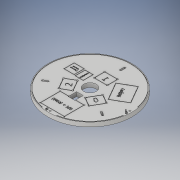
# Autodesk Inventor part: Robot Plate v1.4
Saved by Autodesk Inventor 2019 (Build 230136000, 136)
## iProperties
Created: 2019-02-04
Part Number: Robot Plate v1.4
Material: Generic
Document SubType Name: Modeling
Designer: a1213969
Density: 1 g/cm^3
Appearance: Default
Author: a1213969
Autodesk Inventor part; units mm, degrees
(part 1 of 4)
ref_plane "YZ Plane" through (0, 0, 0) normal (1, 0, 0) x (0, 1, 0)
ref_plane "XZ Plane" through (0, 0, 0) normal (0, 1, 0) x (-1, 0, 0)
ref_plane "XY Plane" through (0, 0, 0) normal (0, 0, 1) x (1, 0, 0)
sketch "Sketch1" plane through (0, 0, 0) normal (0, 1, 0) x (-1, 0, 0)
  circle A0 centre (0, 0) radius 100
  circle A1 centre (0, 0) radius 15
  dimension "d0" = 200
  dimension "d1" = 30
  constraints: 2 centre point, 2 coincident
  measures "d0" diameter of A0
  measures "d1" diameter of A1
extrude "Extrusion1" add sketch "Sketch1" along normal blind 10
sketch "Sketch2" plane through (0, 10, 0) normal (0, 1, 0) x (1, 0, 0)
  circle A0 centre (0, 0) radius 15 construction
  circle A1 centre (0, 0) radius 100 construction
  line L0 (140, 0) -> (-140, 0) construction
  line L1 (0, 140) -> (0, -140) construction
  line L2 (0, 0) -> (0, 38) construction
  line L3 (15, 26) -> (-15, 26) construction
  line L4 (-15, 26) -> (-15, 50) construction
  line L5 (-15, 50) -> (15, 50) construction
  line L6 (15, 50) -> (15, 26) construction
  line L7 (15, 26) -> (-15, 50) construction
  line L8 (-15, 26) -> (15, 50) construction
  dimension "d4" = 38
  dimension "d5" = 30
  dimension "d6" = 24
  constraints: 14 end point, 4 coincident, 2 midpoint, 2 parallel, 1 horizontal, 1 perpendicular, 1 point on line
  measures "d4" distance of L2.start L2.end
  measures "d5" distance of L4.end L5.end
  measures "d6" distance between parallel lines of L3 L5
hole "Hole1" at (15, 10, -50) at (-15, 10, -26) at (-15, 10, -50) at (15, 10, -50) at (-15, 10, -50) at (-15, 10, -26) at (15, 10, -26) direction (0, -1, 0) diameter 4 end through all
pattern_circular "Circular Pattern1" count 3 over 360 about axis through (0, 0, 0) along (0, 1, 0) of "Hole1"
sketch "Sketch3" plane through (0, 10, 0) normal (0, 1, 0) x (1, 0, 0)
  circle A0 centre (30.0167, -0.0096) radius 2 construction
  circle A1 centre (15.0167, -25.9904) radius 2 construction
  circle A2 centre (50.8013, -12.0096) radius 2 construction
  circle A3 centre (35.8013, -37.9904) radius 2 construction
  circle A4 centre (-15.0167, -25.9904) radius 2 construction
  circle A5 centre (-30.0167, -0.0096) radius 2 construction
  circle A6 centre (-35.8013, -37.9904) radius 2 construction
  circle A7 centre (-50.8013, -12.0096) radius 2 construction
  circle A8 centre (-15, 26) radius 2 construction
  circle A9 centre (15, 50) radius 2 construction
  circle A10 centre (-15, 50) radius 2 construction
  circle A11 centre (15, 26) radius 2 construction
  circle A12 centre (0, 0) radius 15 construction
  circle A13 centre (0, 0) radius 100 construction
  circle A14 centre (-15, 50) radius 2 construction
  circle A15 centre (15, 50) radius 2 construction
  line L0 (-15, 50) -> (15, 50) construction
  line L1 (0, 50) -> (0, 100) construction
  circle A16 centre (0, 0) radius 15 construction
  line L2 (0, 0) -> (0, -100) construction
  circle A17 centre (0, 0) radius 100 construction
  line L3 (0, -100) -> (0, -66) construction
  line L4 (-29, -42) -> (29, -42) construction
  line L5 (29, -42) -> (29, -90) construction
  line L6 (29, -90) -> (-29, -90) construction
  line L7 (-29, -90) -> (-29, -42) construction
  line L8 (-29, -42) -> (29, -90) construction
  line L9 (29, -42) -> (-29, -90) construction
  dimension "d17" = 34
  dimension "d18" = 58
  dimension "d19" = 48
  constraints: 20 end point, 4 coincident, 3 midpoint, 2 horizontal, 2 parallel, 2 vertical, 1 perpendicular, 1 point on circle, 1 point on line, 1 vertical alignment, 1 other
  measures "d17" distance of L2.end L3.end
  measures "d18" distance of L5.end L6.end
  measures "d19" distance of L4.end L5.end
hole "Hole2" at (29, 10, 90) at (-29, 10, 90) at (-29, 10, 42) at (29, 10, 42) direction (0, -1, 0) diameter 2.5 end through all
sketch "Sketch4" plane through (0, 10, 0) normal (0, 1, 0) x (1, 0, 0)
  circle A0 centre (-29, -42) radius 1.25 construction
  circle A1 centre (29, -90) radius 1.25 construction
  circle A2 centre (-29, -90) radius 1.25 construction
  circle A3 centre (29, -42) radius 1.25 construction
  circle A4 centre (30.0167, -0.0096) radius 2 construction
  circle A5 centre (15.0167, -25.9904) radius 2 construction
  circle A6 centre (50.8013, -12.0096) radius 2 construction
  circle A7 centre (35.8013, -37.9904) radius 2 construction
  circle A8 centre (-15.0167, -25.9904) radius 2 construction
  circle A9 centre (-30.0167, -0.0096) radius 2 construction
  circle A10 centre (-35.8013, -37.9904) radius 2 construction
  circle A11 centre (-50.8013, -12.0096) radius 2 construction
  circle A12 centre (-15, 26) radius 2 construction
  circle A13 centre (15, 50) radius 2 construction
  circle A14 centre (-15, 50) radius 2 construction
  circle A15 centre (15, 26) radius 2 construction
  circle A16 centre (0, 0) radius 15 construction
  circle A17 centre (0, 0) radius 100 construction
  circle A18 centre (50.8013, -12.0096) radius 2 construction
  circle A19 centre (15, 50) radius 2 construction
  line L0 (50.8013, -12.0096) -> (15, 50) construction
  line L1 (15, 50) -> (49.641, 70) construction
  line L2 (49.641, 70) -> (85.4423, 7.9904) construction
  line L3 (85.4423, 7.9904) -> (50.8013, -12.0096) construction
  line L4 (68.1218, -2.0096) -> (32.3205, 60) construction
  line L5 (68.1218, -2.0096) -> (58.3013, 15) construction
  line L6 (50.2211, 28.9952) -> (62.7211, 7.3446) construction
  line L7 (50.2211, 28.9952) -> (37.7211, 50.6458) construction
  dimension "d27" = 40
  dimension "d28" = 25
  dimension "d29" = 25
  constraints: 16 end point, 3 midpoint, 3 point on line, 2 coincident, 2 parallel, 1 perpendicular
  measures "d27" distance of L0.end L1.end
  measures "d28" distance of L6.start L6.end
  measures "d29" distance of L6.start L7.end
hole "Hole3" at (50.2211, 10, -28.9952) at (62.7211, 10, -7.3446) at (37.7211, 10, -50.6458) direction (0, -1, 0) diameter 2.5 end through all
sketch "Sketch5" plane through (0, 10, 0) normal (0, 1, 0) x (1, 0, 0)
  circle A0 centre (62.7211, 7.3446) radius 1.25 construction
  circle A1 centre (50.2211, 28.9952) radius 1.25 construction
  circle A2 centre (37.7211, 50.6458) radius 1.25 construction
  circle A3 centre (-29, -42) radius 1.25 construction
  circle A4 centre (29, -90) radius 1.25 construction
  circle A5 centre (-29, -90) radius 1.25 construction
  circle A6 centre (29, -42) radius 1.25 construction
  circle A7 centre (30.0167, -0.0096) radius 2 construction
  circle A8 centre (15.0167, -25.9904) radius 2 construction
  circle A9 centre (50.8013, -12.0096) radius 2 construction
  circle A10 centre (35.8013, -37.9904) radius 2 construction
  circle A11 centre (-15.0167, -25.9904) radius 2 construction
  circle A12 centre (-30.0167, -0.0096) radius 2 construction
  circle A13 centre (-35.8013, -37.9904) radius 2 construction
  circle A14 centre (-50.8013, -12.0096) radius 2 construction
  circle A15 centre (-15, 26) radius 2 construction
  circle A16 centre (15, 50) radius 2 construction
  circle A17 centre (-15, 50) radius 2 construction
  circle A18 centre (15, 26) radius 2 construction
  circle A19 centre (0, 0) radius 15 construction
  circle A20 centre (0, 0) radius 100 construction
  circle A21 centre (-50.8013, -12.0096) radius 2 construction
  line L0 (-15, 50) -> (-50.8013, 50) construction
  line L1 (-50.8013, 50) -> (-50.8013, -12.0096) construction
  line L2 (-50.8013, -12.0096) -> (-15, -12.0096) construction
  line L3 (-15, -12.0096) -> (-15, 50) construction
  line L4 (-32.9006, -12.0096) -> (-32.9006, 50) construction
  line L5 (-32.9006, 18.9952) -> (-32.9006, 6.7452) construction
  line L6 (-32.9006, 18.9952) -> (-32.9006, 31.2452) construction
  dimension "d37" = 12.25
  dimension "d38" = 12.25
  constraints: 14 end point, 3 midpoint, 2 coincident, 2 parallel, 2 point on line, 1 horizontal, 1 perpendicular
  measures "d37" distance of L5.start L5.end
  measures "d38" distance of L5.start L6.end
hole "Hole4" at (-32.9006, 10, -6.7452) at (-32.9006, 10, -31.2452) direction (0, -1, 0) diameter 1.6 end through all
sketch "Sketch6" plane through (0, 10, 0) normal (0, 1, 0) x (1, 0, 0)
  circle A0 centre (-32.9006, 6.7452) radius 0.8 construction
  circle A1 centre (-32.9006, 31.2452) radius 0.8 construction
  circle A2 centre (62.7211, 7.3446) radius 1.25 construction
  circle A3 centre (50.2211, 28.9952) radius 1.25 construction
  circle A4 centre (37.7211, 50.6458) radius 1.25 construction
  circle A5 centre (-29, -42) radius 1.25 construction
  circle A6 centre (29, -90) radius 1.25 construction
  circle A7 centre (-29, -90) radius 1.25 construction
  circle A8 centre (29, -42) radius 1.25 construction
  circle A9 centre (30.0167, -0.0096) radius 2 construction
  circle A10 centre (15.0167, -25.9904) radius 2 construction
  circle A11 centre (50.8013, -12.0096) radius 2 construction
  circle A12 centre (35.8013, -37.9904) radius 2 construction
  circle A13 centre (-15.0167, -25.9904) radius 2 construction
  circle A14 centre (-30.0167, -0.0096) radius 2 construction
  circle A15 centre (-35.8013, -37.9904) radius 2 construction
  circle A16 centre (-50.8013, -12.0096) radius 2 construction
  circle A17 centre (-15, 26) radius 2 construction
  circle A18 centre (15, 50) radius 2 construction
  circle A19 centre (-15, 50) radius 2 construction
  circle A20 centre (15, 26) radius 2 construction
  circle A21 centre (0, 0) radius 15 construction
  circle A22 centre (0, 0) radius 100 construction
  circle A23 centre (-29, -42) radius 1.25 construction
  line L0 (29, -90) -> (-29, -90) construction
  line L1 (-29, -90) -> (-29, -42) construction
  line L2 (-29, -42) -> (29, -42) construction
  line L3 (29, -42) -> (29, -90) construction
  circle A24 centre (-32.9006, 6.7452) radius 0.8 construction
  line L4 (-32.9006, 6.7452) -> (-38.9006, 6.7452) construction
  line L5 (-38.9006, 6.7452) -> (-38.9006, 31.2452) construction
  line L6 (-38.9006, 31.2452) -> (-32.9006, 31.2452) construction
  line L7 (-32.9006, 31.2452) -> (-32.9006, 6.7452) construction
  line L8 (-32.9006, 6.7452) -> (-26.9006, 6.7452) construction
  line L9 (-26.9006, 6.7452) -> (-26.9006, 31.2452) construction
  line L10 (-26.9006, 31.2452) -> (-32.9006, 31.2452) construction
  line L11 (-32.9006, 31.2452) -> (-32.9006, 6.7452) construction
  line L12 (-26.9006, 6.7452) -> (-38.9006, 6.7452) construction
  line L13 (-57.6246, 32.9097) -> (-45.6246, 32.9097) construction
  line L14 (-45.6246, 32.9097) -> (-70.6246, 32.9097) construction
  line L15 (-70.6246, 32.9097) -> (-70.6246, 7.9097) construction
  line L16 (-70.6246, 7.9097) -> (-45.6246, 7.9097) construction
  line L17 (-45.6246, 7.9097) -> (-45.6246, 32.9097) construction
  circle A25 centre (62.7211, 7.3446) radius 1.25 construction
  circle A26 centre (37.7211, 50.6458) radius 1.25 construction
  line L18 (62.7211, 7.3446) -> (37.7211, 50.6458) construction
  circle A27 centre (50.8013, -12.0096) radius 2 construction
  circle A28 centre (30.0167, -0.0096) radius 2 construction
  line L19 (50.8013, -12.0096) -> (30.0167, -0.0096) construction
  line L20 (30.0167, -0.0096) -> (15.0167, -25.9904) construction
  line L21 (15.0167, -25.9904) -> (35.8013, -37.9904) construction
  line L22 (35.8013, -37.9904) -> (50.8013, -12.0096) construction
  circle A29 centre (-15.0167, -25.9904) radius 2 construction
  circle A30 centre (-30.0167, -0.0096) radius 2 construction
  line L23 (-15.0167, -25.9904) -> (-30.0167, -0.0096) construction
  line L24 (-30.0167, -0.0096) -> (-50.8013, -12.0096) construction
  line L25 (-50.8013, -12.0096) -> (-35.8013, -37.9904) construction
  line L26 (-35.8013, -37.9904) -> (-15.0167, -25.9904) construction
  circle A31 centre (15, 26) radius 2 construction
  line L27 (15, 26) -> (-15, 26) construction
  line L28 (-15, 26) -> (-15, 50) construction
  line L29 (-15, 50) -> (15, 50) construction
  line L30 (15, 50) -> (15, 26) construction
  spline S0 degree 2 poles (30.1224, -21.8265) (27.3264, -20.2123) (25.6457, -17.0748) (26.623, -15.382) knots 0 0 0 1 2 2 2
  spline S1 degree 2 poles (26.623, -15.382) (27.6149, -13.664) (31.2132, -13.5968) (33.9502, -15.177) knots 0 0 0 1 2 2 2
  spline S2 degree 2 poles (33.9502, -15.177) (36.7631, -16.801) (38.4269, -19.9288) (37.4448, -21.63) knots 0 0 0 1 2 2 2
  spline S3 degree 2 poles (37.4448, -21.63) (36.4577, -23.3396) (32.8341, -23.3922) (30.1224, -21.8265) knots 0 0 0 1 2 2 2
  spline S4 degree 2 poles (27.9866, -18.213) (28.3836, -18.7117) (29.8697, -19.7942) (30.9392, -20.4117) knots 0 0 0 1 2 2 2
  spline S5 degree 2 poles (30.9392, -20.4117) (32.0088, -21.0292) (33.6809, -21.77) (34.333, -21.8658) knots 0 0 0 1 2 2 2
  spline S6 degree 2 poles (34.333, -21.8658) (34.9851, -21.9616) (35.9555, -21.5449) (36.291, -20.9639) knots 0 0 0 1 2 2 2
  spline S7 degree 2 poles (36.291, -20.9639) (36.6265, -20.3828) (36.5118, -19.3172) (36.0908, -18.7822) knots 0 0 0 1 2 2 2
  spline S8 degree 2 poles (36.0908, -18.7822) (35.6818, -18.2653) (34.1524, -17.1802) (33.1334, -16.5918) knots 0 0 0 1 2 2 2
  spline S9 degree 2 poles (33.1334, -16.5918) (32.0386, -15.9598) (30.4954, -15.2485) (29.7963, -15.1368) knots 0 0 0 1 2 2 2
  spline S10 degree 2 poles (29.7963, -15.1368) (29.1406, -15.0277) (28.1268, -15.4418) (27.7767, -16.0481) knots 0 0 0 1 2 2 2
  spline S11 degree 2 poles (27.7767, -16.0481) (27.4461, -16.6208) (27.5608, -17.6864) (27.9866, -18.213) knots 0 0 0 1 2 2 2
  line L31 (17.9317, -63) -> (18.9846, -63)
  line L32 (18.9846, -63) -> (20.9125, -65.4271)
  line L33 (20.9125, -65.4271) -> (21.8419, -65.4271)
  line L34 (21.8419, -65.4271) -> (21.8419, -63)
  line L35 (21.8419, -63) -> (22.6526, -63)
  line L36 (22.6526, -63) -> (22.6526, -69.1)
  line L37 (22.6526, -69.1) -> (21.0806, -69.1)
  spline S12 degree 2 poles (21.0806, -69.1) (20.5566, -69.1) (19.8497, -68.9863) (19.5284, -68.7787) knots 0 0 0 1 2 2 2
  spline S13 degree 2 poles (19.5284, -68.7787) (19.2071, -68.5711) (18.8363, -67.9235) (18.8363, -67.444) knots 0 0 0 1 2 2 2
  spline S14 degree 2 poles (18.8363, -67.444) (18.8363, -66.7767) (19.5185, -65.872) (20.1018, -65.6545) knots 0 0 0 1 2 2 2
  line L38 (20.1018, -65.6545) -> (17.9317, -63)
  spline S15 degree 2 poles (19.6816, -67.3797) (19.6816, -67.6467) (19.8695, -68.057) (20.0672, -68.1904) knots 0 0 0 1 2 2 2
  spline S16 degree 2 poles (20.0672, -68.1904) (20.2402, -68.3041) (20.7, -68.3981) (21.0361, -68.3981) knots 0 0 0 1 2 2 2
  line L39 (21.0361, -68.3981) -> (21.8419, -68.3981)
  line L40 (21.8419, -68.3981) -> (21.8419, -66.1044)
  line L41 (21.8419, -66.1044) -> (21.13, -66.1044)
  spline S17 degree 2 poles (21.13, -66.1044) (20.7791, -66.1044) (20.2205, -66.228) (20.0277, -66.4207) knots 0 0 0 1 2 2 2
  spline S18 degree 2 poles (20.0277, -66.4207) (19.8497, -66.5888) (19.6816, -67.0634) (19.6816, -67.3797) knots 0 0 0 1 2 2 2
  spline S19 degree 2 poles (13.5915, -67.2611) (13.5915, -66.8656) (13.8733, -66.1538) (14.1254, -65.9066) knots 0 0 0 1 2 2 2
  spline S20 degree 2 poles (14.1254, -65.9066) (14.4418, -65.5952) (15.297, -65.2739) (15.9495, -65.2739) knots 0 0 0 1 2 2 2
  line L42 (15.9495, -65.2739) -> (16.6366, -65.2739)
  line L43 (16.6366, -65.2739) -> (16.6366, -63)
  line L44 (16.6366, -63) -> (17.4473, -63)
  line L45 (17.4473, -63) -> (17.4473, -69.1)
  line L46 (17.4473, -69.1) -> (15.9149, -69.1)
  spline S21 degree 2 poles (15.9149, -69.1) (15.3711, -69.1) (14.6098, -68.922) (14.3182, -68.7194) knots 0 0 0 1 2 2 2
  spline S22 degree 2 poles (14.3182, -68.7194) (13.9771, -68.487) (13.5915, -67.7703) (13.5915, -67.2611) knots 0 0 0 1 2 2 2
  spline S23 degree 2 poles (14.4368, -67.2364) (14.4368, -67.5528) (14.6543, -68.0174) (14.8768, -68.1657) knots 0 0 0 1 2 2 2
  spline S24 degree 2 poles (14.8768, -68.1657) (15.0696, -68.2942) (15.5837, -68.3981) (15.9643, -68.3981) knots 0 0 0 1 2 2 2
  line L47 (15.9643, -68.3981) -> (16.6366, -68.3981)
  line L48 (16.6366, -68.3981) -> (16.6366, -65.966)
  line L49 (16.6366, -65.966) -> (16.0829, -65.966)
  spline S25 degree 2 poles (16.0829, -65.966) (15.5886, -65.966) (14.9806, -66.1241) (14.7829, -66.3318) knots 0 0 0 1 2 2 2
  spline S26 degree 2 poles (14.7829, -66.3318) (14.6, -66.5147) (14.4368, -66.9447) (14.4368, -67.2364) knots 0 0 0 1 2 2 2
  line L50 (10.6948, -63) -> (13.0577, -63)
  line L51 (13.0577, -63) -> (13.0577, -63.6229)
  line L52 (13.0577, -63.6229) -> (12.2816, -63.6229)
  line L53 (12.2816, -63.6229) -> (12.2816, -68.4771)
  line L54 (12.2816, -68.4771) -> (13.0577, -68.4771)
  line L55 (13.0577, -68.4771) -> (13.0577, -69.1)
  line L56 (13.0577, -69.1) -> (10.6948, -69.1)
  line L57 (10.6948, -69.1) -> (10.6948, -68.4771)
  line L58 (10.6948, -68.4771) -> (11.4709, -68.4771)
  line L59 (11.4709, -68.4771) -> (11.4709, -63.6229)
  line L60 (11.4709, -63.6229) -> (10.6948, -63.6229)
  line L61 (10.6948, -63.6229) -> (10.6948, -63)
  line L62 (2.2269, -65.3431) -> (4.2932, -65.3431)
  line L63 (4.2932, -65.3431) -> (4.2932, -63.2768)
  line L64 (4.2932, -63.2768) -> (4.9754, -63.2768)
  line L65 (4.9754, -63.2768) -> (4.9754, -65.3431)
  line L66 (4.9754, -65.3431) -> (7.0417, -65.3431)
  line L67 (7.0417, -65.3431) -> (7.0417, -66.0006)
  line L68 (7.0417, -66.0006) -> (4.9754, -66.0006)
  line L69 (4.9754, -66.0006) -> (4.9754, -68.0669)
  line L70 (4.9754, -68.0669) -> (4.2932, -68.0669)
  line L71 (4.2932, -68.0669) -> (4.2932, -66.0006)
  line L72 (4.2932, -66.0006) -> (2.2269, -66.0006)
  line L73 (2.2269, -66.0006) -> (2.2269, -65.3431)
  spline S27 degree 2 poles (-3.354, -62.8912) (-2.6916, -62.8912) (-1.7623, -63.1681) (-1.352, -63.3658) knots 0 0 0 1 2 2 2
  line L74 (-1.352, -63.3658) -> (-1.352, -64.3841)
  line L75 (-1.352, -64.3841) -> (-1.4113, -64.3841)
  spline S28 degree 2 poles (-1.4113, -64.3841) (-1.8117, -64.0084) (-2.8251, -63.5932) (-3.2947, -63.5932) knots 0 0 0 1 2 2 2
  spline S29 degree 2 poles (-3.2947, -63.5932) (-3.967, -63.5932) (-4.6541, -64.1518) (-4.6541, -64.6115) knots 0 0 0 1 2 2 2
  spline S30 degree 2 poles (-4.6541, -64.6115) (-4.6541, -64.9773) (-4.2932, -65.4321) (-3.9027, -65.5458) knots 0 0 0 1 2 2 2
  spline S31 degree 2 poles (-3.9027, -65.5458) (-3.6209, -65.6249) (-3.1513, -65.7336) (-2.8004, -65.8226) knots 0 0 0 1 2 2 2
  spline S32 degree 2 poles (-2.8004, -65.8226) (-2.484, -65.9066) (-1.9847, -66.1588) (-1.7919, -66.3614) knots 0 0 0 1 2 2 2
  spline S33 degree 2 poles (-1.7919, -66.3614) (-1.6041, -66.5641) (-1.3965, -67.1079) (-1.3965, -67.4638) knots 0 0 0 1 2 2 2
  spline S34 degree 2 poles (-1.3965, -67.4638) (-1.3965, -68.2053) (-2.5532, -69.2088) (-3.4479, -69.2088) knots 0 0 0 1 2 2 2
  spline S35 degree 2 poles (-3.4479, -69.2088) (-3.962, -69.2088) (-4.8716, -69.0061) (-5.2621, -68.8133) knots 0 0 0 1 2 2 2
  line L76 (-5.2621, -68.8133) -> (-5.2621, -67.8444)
  line L77 (-5.2621, -67.8444) -> (-5.2028, -67.8444)
  spline S36 degree 2 poles (-5.2028, -67.8444) (-4.9111, -68.1113) (-4.0016, -68.5068) (-3.5023, -68.5068) knots 0 0 0 1 2 2 2
  spline S37 degree 2 poles (-3.5023, -68.5068) (-2.9388, -68.5068) (-2.2418, -67.9779) (-2.2418, -67.5478) knots 0 0 0 1 2 2 2
  spline S38 degree 2 poles (-2.2418, -67.5478) (-2.2418, -67.1622) (-2.6521, -66.7025) (-3.0376, -66.5987) knots 0 0 0 1 2 2 2
  spline S39 degree 2 poles (-3.0376, -66.5987) (-3.2947, -66.5295) (-4.0411, -66.3515) (-4.2883, -66.2774) knots 0 0 0 1 2 2 2
  spline S40 degree 2 poles (-4.2883, -66.2774) (-4.9161, -66.0846) (-5.4994, -65.3085) (-5.4994, -64.74) knots 0 0 0 1 2 2 2
  spline S41 degree 2 poles (-5.4994, -64.74) (-5.4994, -64.3792) (-5.2077, -63.6871) (-4.9457, -63.4449) knots 0 0 0 1 2 2 2
  spline S42 degree 2 poles (-4.9457, -63.4449) (-4.6541, -63.178) (-3.9126, -62.8912) (-3.354, -62.8912) knots 0 0 0 1 2 2 2
  line L78 (-9.8594, -63) -> (-9.0882, -63)
  line L79 (-9.0882, -63) -> (-9.0882, -65.61)
  spline S43 degree 2 poles (-9.0882, -65.61) (-9.0882, -65.9264) (-9.0289, -66.4702) (-8.9399, -66.6333) knots 0 0 0 1 2 2 2
  spline S44 degree 2 poles (-8.9399, -66.6333) (-8.846, -66.8063) (-8.5098, -66.9744) (-8.2231, -66.9744) knots 0 0 0 1 2 2 2
  spline S45 degree 2 poles (-8.2231, -66.9744) (-7.9364, -66.9744) (-7.3284, -66.6679) (-7.0368, -66.4207) knots 0 0 0 1 2 2 2
  line L80 (-7.0368, -66.4207) -> (-7.0368, -63)
  line L81 (-7.0368, -63) -> (-6.2656, -63)
  line L82 (-6.2656, -63) -> (-6.2656, -69.3719)
  line L83 (-6.2656, -69.3719) -> (-7.0368, -69.3719)
  line L84 (-7.0368, -69.3719) -> (-7.0368, -67.0683)
  spline S46 degree 2 poles (-7.0368, -67.0683) (-7.3828, -67.3797) (-8.0501, -67.706) (-8.4258, -67.706) knots 0 0 0 1 2 2 2
  spline S47 degree 2 poles (-8.4258, -67.706) (-9.0981, -67.706) (-9.8594, -66.8162) (-9.8594, -65.9709) knots 0 0 0 1 2 2 2
  line L85 (-9.8594, -65.9709) -> (-9.8594, -63)
  line L86 (-11.7279, -63) -> (-10.9568, -63)
  line L87 (-10.9568, -63) -> (-10.9568, -67.5775)
  line L88 (-10.9568, -67.5775) -> (-11.7279, -67.5775)
  line L89 (-11.7279, -67.5775) -> (-11.7279, -63)
  line L90 (-11.7823, -68.3387) -> (-10.9073, -68.3387)
  line L91 (-10.9073, -68.3387) -> (-10.9073, -69.1395)
  line L92 (-10.9073, -69.1395) -> (-11.7823, -69.1395)
  line L93 (-11.7823, -69.1395) -> (-11.7823, -68.3387)
  spline S48 degree 2 poles (-14.8471, -62.8962) (-13.7497, -62.8962) (-12.5436, -64.1271) (-12.5436, -65.264) knots 0 0 0 1 2 2 2
  spline S49 degree 2 poles (-12.5436, -65.264) (-12.5436, -66.3812) (-13.7151, -67.706) (-14.6593, -67.706) knots 0 0 0 1 2 2 2
  spline S50 degree 2 poles (-14.6593, -67.706) (-15.0844, -67.706) (-15.7419, -67.4588) (-15.9841, -67.1968) knots 0 0 0 1 2 2 2
  spline S51 degree 2 poles (-15.9841, -67.1968) (-16.2312, -66.9348) (-16.4932, -66.1785) (-16.4932, -65.6298) knots 0 0 0 1 2 2 2
  line L94 (-16.4932, -65.6298) -> (-16.4932, -65.2096)
  line L95 (-16.4932, -65.2096) -> (-13.3246, -65.2096)
  spline S52 degree 2 poles (-13.3246, -65.2096) (-13.3246, -64.4138) (-14.1254, -63.5685) (-14.8372, -63.5685) knots 0 0 0 1 2 2 2
  spline S53 degree 2 poles (-14.8372, -63.5685) (-15.0893, -63.5685) (-15.5787, -63.6822) (-15.7765, -63.7712) knots 0 0 0 1 2 2 2
  spline S54 degree 2 poles (-15.7765, -63.7712) (-15.9841, -63.87) (-16.2708, -64.043) (-16.3647, -64.1221) knots 0 0 0 1 2 2 2
  line L96 (-16.3647, -64.1221) -> (-16.4092, -64.1221)
  line L97 (-16.4092, -64.1221) -> (-16.4092, -63.2818)
  spline S55 degree 2 poles (-16.4092, -63.2818) (-16.2757, -63.2274) (-15.8704, -63.0692) (-15.7122, -63.0247) knots 0 0 0 1 2 2 2
  spline S56 degree 2 poles (-15.7122, -63.0247) (-15.4897, -62.9605) (-15.1239, -62.8962) (-14.8471, -62.8962) knots 0 0 0 1 2 2 2
  spline S57 degree 2 poles (-15.7419, -65.7979) (-15.732, -66.1093) (-15.6034, -66.5641) (-15.4799, -66.7173) knots 0 0 0 1 2 2 2
  spline S58 degree 2 poles (-15.4799, -66.7173) (-15.3464, -66.8904) (-14.9262, -67.0733) (-14.6148, -67.0733) knots 0 0 0 1 2 2 2
  spline S59 degree 2 poles (-14.6148, -67.0733) (-14.3083, -67.0733) (-13.8782, -66.8904) (-13.7003, -66.7124) knots 0 0 0 1 2 2 2
  spline S60 degree 2 poles (-13.7003, -66.7124) (-13.5273, -66.5295) (-13.3493, -66.0895) (-13.3246, -65.7979) knots 0 0 0 1 2 2 2
  line L98 (-13.3246, -65.7979) -> (-15.7419, -65.7979)
  line L99 (-18.0603, -63) -> (-17.2891, -63)
  line L100 (-17.2891, -63) -> (-17.2891, -69.3719)
  line L101 (-17.2891, -69.3719) -> (-18.0603, -69.3719)
  line L102 (-18.0603, -69.3719) -> (-18.0603, -63)
  line L103 (-22.7119, -63) -> (-21.9407, -63)
  line L104 (-21.9407, -63) -> (-21.9407, -63.4647)
  spline S61 degree 2 poles (-21.9407, -63.4647) (-21.7628, -63.3164) (-21.5008, -63.1186) (-21.3228, -63.0346) knots 0 0 0 1 2 2 2
  spline S62 degree 2 poles (-21.3228, -63.0346) (-21.1597, -62.9555) (-20.8087, -62.8715) (-20.5764, -62.8715) knots 0 0 0 1 2 2 2
  spline S63 degree 2 poles (-20.5764, -62.8715) (-20.2007, -62.8715) (-19.568, -63.1829) (-19.3455, -63.4844) knots 0 0 0 1 2 2 2
  spline S64 degree 2 poles (-19.3455, -63.4844) (-19.1231, -63.786) (-18.8759, -64.6758) (-18.8759, -65.2541) knots 0 0 0 1 2 2 2
  spline S65 degree 2 poles (-18.8759, -65.2541) (-18.8759, -65.8572) (-19.1873, -66.7371) (-19.4592, -67.0683) knots 0 0 0 1 2 2 2
  spline S66 degree 2 poles (-19.4592, -67.0683) (-19.7113, -67.3649) (-20.4182, -67.706) (-20.8087, -67.706) knots 0 0 0 1 2 2 2
  spline S67 degree 2 poles (-20.8087, -67.706) (-21.1498, -67.706) (-21.659, -67.5528) (-21.9407, -67.3946) knots 0 0 0 1 2 2 2
  line L105 (-21.9407, -67.3946) -> (-21.9407, -69.3719)
  line L106 (-21.9407, -69.3719) -> (-22.7119, -69.3719)
  line L107 (-22.7119, -69.3719) -> (-22.7119, -63)
  line L108 (-21.9407, -64.1122) -> (-21.9407, -66.7569)
  spline S68 degree 2 poles (-21.9407, -66.7569) (-21.654, -66.8953) (-21.1992, -66.9991) (-20.9372, -66.9991) knots 0 0 0 1 2 2 2
  spline S69 degree 2 poles (-20.9372, -66.9991) (-20.344, -66.9991) (-19.6718, -66.1093) (-19.6718, -65.269) knots 0 0 0 1 2 2 2
  spline S70 degree 2 poles (-19.6718, -65.269) (-19.6718, -64.4583) (-20.1859, -63.6031) (-20.7543, -63.6031) knots 0 0 0 1 2 2 2
  spline S71 degree 2 poles (-20.7543, -63.6031) (-21.0559, -63.6031) (-21.6688, -63.8799) (-21.9407, -64.1122) knots 0 0 0 1 2 2 2
  line L109 (-28.7333, -12.2324) -> (-25.0332, -18.6413)
  line L110 (-25.0332, -18.6413) -> (-26.507, -19.4922)
  spline S72 degree 2 poles (-26.507, -19.4922) (-27.5541, -19.176) (-29.4683, -18.6417) (-30.4571, -18.4266) knots 0 0 0 1 2 2 2
  spline S73 degree 2 poles (-30.4571, -18.4266) (-32.4481, -17.9928) (-34.5153, -18.0297) (-35.349, -18.5111) knots 0 0 0 1 2 2 2
  spline S74 degree 2 poles (-35.349, -18.5111) (-35.787, -18.7639) (-36.2883, -19.4127) (-36.3578, -19.7785) knots 0 0 0 1 2 2 2
  spline S75 degree 2 poles (-36.3578, -19.7785) (-36.4273, -20.1443) (-36.2683, -20.9059) (-36.0447, -21.2932) knots 0 0 0 1 2 2 2
  spline S76 degree 2 poles (-36.0447, -21.2932) (-35.8307, -21.6638) (-35.2079, -22.3148) (-34.8653, -22.5774) knots 0 0 0 1 2 2 2
  spline S77 degree 2 poles (-34.8653, -22.5774) (-34.5773, -22.8041) (-33.9244, -23.157) (-33.7092, -23.2574) knots 0 0 0 1 2 2 2
  line L111 (-33.7092, -23.2574) -> (-33.6654, -23.3332)
  line L112 (-33.6654, -23.3332) -> (-35.1477, -24.1889)
  spline S78 degree 2 poles (-35.1477, -24.1889) (-35.6062, -23.881) (-36.9086, -22.5781) (-37.3073, -21.8875) knots 0 0 0 1 2 2 2
  spline S79 degree 2 poles (-37.3073, -21.8875) (-38.1485, -20.4305) (-37.5555, -17.8985) (-36.2417, -17.14) knots 0 0 0 1 2 2 2
  spline S80 degree 2 poles (-36.2417, -17.14) (-35.6269, -16.7851) (-34.4342, -16.4782) (-33.8504, -16.478) knots 0 0 0 1 2 2 2
  spline S81 degree 2 poles (-33.8504, -16.478) (-33.2497, -16.4681) (-31.934, -16.6854) (-31.2711, -16.8417) knots 0 0 0 1 2 2 2
  spline S82 degree 2 poles (-31.2711, -16.8417) (-30.176, -17.0853) (-27.7146, -17.8089) (-26.9911, -18.0312) knots 0 0 0 1 2 2 2
  line L113 (-26.9911, -18.0312) -> (-29.9376, -12.9277)
  line L114 (-29.9376, -12.9277) -> (-28.7333, -12.2324)
  line L115 (-31.4006, 11.8371) -> (-31.4006, 11.432)
  line L116 (-31.4006, 11.432) -> (-34.0263, 11.432)
  line L117 (-34.0263, 11.432) -> (-32.2404, 10.6367)
  line L118 (-32.2404, 10.6367) -> (-32.2404, 10.3897)
  line L119 (-32.2404, 10.3897) -> (-34.0263, 9.6017)
  line L120 (-34.0263, 9.6017) -> (-31.4006, 9.6017)
  line L121 (-31.4006, 9.6017) -> (-31.4006, 9.2238)
  line L122 (-31.4006, 9.2238) -> (-34.4486, 9.2238)
  line L123 (-34.4486, 9.2238) -> (-34.4486, 9.7771)
  line L124 (-34.4486, 9.7771) -> (-32.7517, 10.5379)
  line L125 (-32.7517, 10.5379) -> (-34.4486, 11.2739)
  line L126 (-34.4486, 11.2739) -> (-34.4486, 11.8371)
  line L127 (-34.4486, 11.8371) -> (-31.4006, 11.8371)
  line L128 (-31.4006, 14.2034) -> (-31.4006, 13.818)
  line L129 (-31.4006, 13.818) -> (-31.6526, 13.818)
  spline S83 degree 2 poles (-31.6526, 13.818) (-31.497, 13.6402) (-31.3364, 13.3216) (-31.3364, 13.124) knots 0 0 0 1 2 2 2
  spline S84 degree 2 poles (-31.3364, 13.124) (-31.3364, 12.9758) (-31.4352, 12.7115) (-31.5414, 12.6151) knots 0 0 0 1 2 2 2
  spline S85 degree 2 poles (-31.5414, 12.6151) (-31.6476, 12.5163) (-31.9712, 12.4077) (-32.2034, 12.4077) knots 0 0 0 1 2 2 2
  line L130 (-32.2034, 12.4077) -> (-33.6879, 12.4077)
  line L131 (-33.6879, 12.4077) -> (-33.6879, 12.793)
  line L132 (-33.6879, 12.793) -> (-32.3837, 12.793)
  spline S86 degree 2 poles (-32.3837, 12.793) (-32.2009, 12.793) (-31.9613, 12.8202) (-31.8724, 12.8671) knots 0 0 0 1 2 2 2
  spline S87 degree 2 poles (-31.8724, 12.8671) (-31.7835, 12.914) (-31.702, 13.0746) (-31.702, 13.2252) knots 0 0 0 1 2 2 2
  spline S88 degree 2 poles (-31.702, 13.2252) (-31.702, 13.366) (-31.8625, 13.6847) (-31.9786, 13.818) knots 0 0 0 1 2 2 2
  line L133 (-31.9786, 13.818) -> (-33.6879, 13.818)
  line L134 (-33.6879, 13.818) -> (-33.6879, 14.2034)
  line L135 (-33.6879, 14.2034) -> (-31.4006, 14.2034)
  line L136 (-31.4006, 15.1543) -> (-31.4006, 14.769)
  line L137 (-31.4006, 14.769) -> (-34.5845, 14.769)
  line L138 (-34.5845, 14.769) -> (-34.5845, 15.1543)
  line L139 (-34.5845, 15.1543) -> (-31.4006, 15.1543)
  spline S89 degree 2 poles (-31.3562, 16.4116) (-31.3562, 16.0979) (-31.7143, 15.7446) (-32.1021, 15.7446) knots 0 0 0 1 2 2 2
  line L140 (-32.1021, 15.7446) -> (-33.3692, 15.7446)
  line L141 (-33.3692, 15.7446) -> (-33.3692, 15.4853)
  line L142 (-33.3692, 15.4853) -> (-33.6879, 15.4853)
  line L143 (-33.6879, 15.4853) -> (-33.6879, 15.7446)
  line L144 (-33.6879, 15.7446) -> (-34.3449, 15.7446)
  line L145 (-34.3449, 15.7446) -> (-34.3449, 16.13)
  line L146 (-34.3449, 16.13) -> (-33.6879, 16.13)
  line L147 (-33.6879, 16.13) -> (-33.6879, 16.8389)
  line L148 (-33.6879, 16.8389) -> (-33.3692, 16.8389)
  line L149 (-33.3692, 16.8389) -> (-33.3692, 16.13)
  line L150 (-33.3692, 16.13) -> (-32.28, 16.13)
  spline S90 degree 2 poles (-32.28, 16.13) (-32.1071, 16.13) (-31.9169, 16.1423) (-31.8354, 16.1843) knots 0 0 0 1 2 2 2
  spline S91 degree 2 poles (-31.8354, 16.1843) (-31.7637, 16.2189) (-31.6921, 16.3745) (-31.6921, 16.5079) knots 0 0 0 1 2 2 2
  spline S92 degree 2 poles (-31.6921, 16.5079) (-31.6921, 16.6017) (-31.7489, 16.7771) (-31.7662, 16.8166) knots 0 0 0 1 2 2 2
  line L151 (-31.7662, 16.8166) -> (-31.7662, 16.8389)
  line L152 (-31.7662, 16.8389) -> (-31.4204, 16.8389)
  spline S93 degree 2 poles (-31.4204, 16.8389) (-31.3908, 16.7302) (-31.3562, 16.5079) (-31.3562, 16.4116) knots 0 0 0 1 2 2 2
  line L153 (-31.4006, 17.5157) -> (-31.4006, 17.1303)
  line L154 (-31.4006, 17.1303) -> (-33.6879, 17.1303)
  line L155 (-33.6879, 17.1303) -> (-33.6879, 17.5157)
  line L156 (-33.6879, 17.5157) -> (-31.4006, 17.5157)
  line L157 (-34.0683, 17.5428) -> (-34.0683, 17.1056)
  line L158 (-34.0683, 17.1056) -> (-34.4684, 17.1056)
  line L159 (-34.4684, 17.1056) -> (-34.4684, 17.5428)
  line L160 (-34.4684, 17.5428) -> (-34.0683, 17.5428)
  spline S94 degree 2 poles (-32.606, 19.998) (-32.033, 19.998) (-31.3562, 19.4521) (-31.3562, 19.0347) knots 0 0 0 1 2 2 2
  spline S95 degree 2 poles (-31.3562, 19.0347) (-31.3562, 18.8643) (-31.4352, 18.6025) (-31.5167, 18.4666) knots 0 0 0 1 2 2 2
  line L161 (-31.5167, 18.4666) -> (-30.5584, 18.4666)
  line L162 (-30.5584, 18.4666) -> (-30.5584, 18.0813)
  line L163 (-30.5584, 18.0813) -> (-33.6879, 18.0813)
  line L164 (-33.6879, 18.0813) -> (-33.6879, 18.4666)
  line L165 (-33.6879, 18.4666) -> (-33.4483, 18.4666)
  spline S96 degree 2 poles (-33.4483, 18.4666) (-33.5792, 18.6099) (-33.7521, 18.9606) (-33.7521, 19.1656) knots 0 0 0 1 2 2 2
  spline S97 degree 2 poles (-33.7521, 19.1656) (-33.7521, 19.5584) (-33.1296, 19.998) (-32.606, 19.998) knots 0 0 0 1 2 2 2
  spline S98 degree 2 poles (-32.5615, 19.6003) (-32.9543, 19.6003) (-33.3865, 19.3509) (-33.3865, 19.0718) knots 0 0 0 1 2 2 2
  spline S99 degree 2 poles (-33.3865, 19.0718) (-33.3865, 18.9087) (-33.2408, 18.6025) (-33.1272, 18.4666) knots 0 0 0 1 2 2 2
  line L166 (-33.1272, 18.4666) -> (-31.8279, 18.4666)
  spline S100 degree 2 poles (-31.8279, 18.4666) (-31.7563, 18.6173) (-31.702, 18.8322) (-31.702, 18.9705) knots 0 0 0 1 2 2 2
  spline S101 degree 2 poles (-31.702, 18.9705) (-31.702, 19.2694) (-32.1416, 19.6003) (-32.5615, 19.6003) knots 0 0 0 1 2 2 2
  line L167 (-31.4006, 20.7909) -> (-31.4006, 20.4056)
  line L168 (-31.4006, 20.4056) -> (-34.5845, 20.4056)
  line L169 (-34.5845, 20.4056) -> (-34.5845, 20.7909)
  line L170 (-34.5845, 20.7909) -> (-31.4006, 20.7909)
  spline S102 degree 2 poles (-31.3488, 22.3495) (-31.3488, 21.8011) (-31.9638, 21.1984) (-32.5319, 21.1984) knots 0 0 0 1 2 2 2
  spline S103 degree 2 poles (-32.5319, 21.1984) (-33.0901, 21.1984) (-33.7521, 21.7838) (-33.7521, 22.2556) knots 0 0 0 1 2 2 2
  spline S104 degree 2 poles (-33.7521, 22.2556) (-33.7521, 22.468) (-33.6286, 22.7965) (-33.4977, 22.9176) knots 0 0 0 1 2 2 2
  spline S105 degree 2 poles (-33.4977, 22.9176) (-33.3668, 23.0411) (-32.9889, 23.172) (-32.7147, 23.172) knots 0 0 0 1 2 2 2
  line L171 (-32.7147, 23.172) -> (-32.5047, 23.172)
  line L172 (-32.5047, 23.172) -> (-32.5047, 21.5887)
  spline S106 degree 2 poles (-32.5047, 21.5887) (-32.1071, 21.5887) (-31.6847, 21.9889) (-31.6847, 22.3445) knots 0 0 0 1 2 2 2
  spline S107 degree 2 poles (-31.6847, 22.3445) (-31.6847, 22.4705) (-31.7415, 22.715) (-31.786, 22.8138) knots 0 0 0 1 2 2 2
  spline S108 degree 2 poles (-31.786, 22.8138) (-31.8354, 22.9176) (-31.9218, 23.0608) (-31.9613, 23.1078) knots 0 0 0 1 2 2 2
  line L173 (-31.9613, 23.1078) -> (-31.9613, 23.13)
  line L174 (-31.9613, 23.13) -> (-31.5414, 23.13)
  spline S109 degree 2 poles (-31.5414, 23.13) (-31.5143, 23.0633) (-31.4352, 22.8608) (-31.413, 22.7817) knots 0 0 0 1 2 2 2
  spline S110 degree 2 poles (-31.413, 22.7817) (-31.3809, 22.6706) (-31.3488, 22.4878) (-31.3488, 22.3495) knots 0 0 0 1 2 2 2
  spline S111 degree 2 poles (-32.7987, 22.7965) (-32.9543, 22.7916) (-33.1815, 22.7274) (-33.2581, 22.6656) knots 0 0 0 1 2 2 2
  spline S112 degree 2 poles (-33.2581, 22.6656) (-33.3445, 22.5989) (-33.4359, 22.389) (-33.4359, 22.2334) knots 0 0 0 1 2 2 2
  spline S113 degree 2 poles (-33.4359, 22.2334) (-33.4359, 22.0802) (-33.3445, 21.8653) (-33.2556, 21.7764) knots 0 0 0 1 2 2 2
  spline S114 degree 2 poles (-33.2556, 21.7764) (-33.1642, 21.69) (-32.9444, 21.6011) (-32.7987, 21.5887) knots 0 0 0 1 2 2 2
  line L175 (-32.7987, 21.5887) -> (-32.7987, 22.7965)
  line L176 (-31.4006, 25.3382) -> (-31.4006, 24.8664)
  line L177 (-31.4006, 24.8664) -> (-32.2602, 24.3107)
  line L178 (-32.2602, 24.3107) -> (-31.4006, 23.7401)
  line L179 (-31.4006, 23.7401) -> (-31.4006, 23.3029)
  line L180 (-31.4006, 23.3029) -> (-32.5344, 24.0958)
  line L181 (-32.5344, 24.0958) -> (-33.6879, 23.3103)
  line L182 (-33.6879, 23.3103) -> (-33.6879, 23.7821)
  line L183 (-33.6879, 23.7821) -> (-32.8357, 24.3354)
  line L184 (-32.8357, 24.3354) -> (-33.6879, 24.901)
  line L185 (-33.6879, 24.901) -> (-33.6879, 25.3382)
  line L186 (-33.6879, 25.3382) -> (-32.5591, 24.5503)
  line L187 (-32.5591, 24.5503) -> (-31.4006, 25.3382)
  spline S115 degree 2 poles (-31.3488, 26.63) (-31.3488, 26.0817) (-31.9638, 25.479) (-32.5319, 25.479) knots 0 0 0 1 2 2 2
  spline S116 degree 2 poles (-32.5319, 25.479) (-33.0901, 25.479) (-33.7521, 26.0644) (-33.7521, 26.5361) knots 0 0 0 1 2 2 2
  spline S117 degree 2 poles (-33.7521, 26.5361) (-33.7521, 26.7486) (-33.6286, 27.0771) (-33.4977, 27.1981) knots 0 0 0 1 2 2 2
  spline S118 degree 2 poles (-33.4977, 27.1981) (-33.3668, 27.3216) (-32.9889, 27.4525) (-32.7147, 27.4525) knots 0 0 0 1 2 2 2
  line L188 (-32.7147, 27.4525) -> (-32.5047, 27.4525)
  line L189 (-32.5047, 27.4525) -> (-32.5047, 25.8692)
  spline S119 degree 2 poles (-32.5047, 25.8692) (-32.1071, 25.8692) (-31.6847, 26.2694) (-31.6847, 26.6251) knots 0 0 0 1 2 2 2
  spline S120 degree 2 poles (-31.6847, 26.6251) (-31.6847, 26.751) (-31.7415, 26.9956) (-31.786, 27.0944) knots 0 0 0 1 2 2 2
  spline S121 degree 2 poles (-31.786, 27.0944) (-31.8354, 27.1981) (-31.9218, 27.3414) (-31.9613, 27.3883) knots 0 0 0 1 2 2 2
  line L190 (-31.9613, 27.3883) -> (-31.9613, 27.4105)
  line L191 (-31.9613, 27.4105) -> (-31.5414, 27.4105)
  spline S122 degree 2 poles (-31.5414, 27.4105) (-31.5143, 27.3438) (-31.4352, 27.1413) (-31.413, 27.0623) knots 0 0 0 1 2 2 2
  spline S123 degree 2 poles (-31.413, 27.0623) (-31.3809, 26.9511) (-31.3488, 26.7683) (-31.3488, 26.63) knots 0 0 0 1 2 2 2
  spline S124 degree 2 poles (-32.7987, 27.0771) (-32.9543, 27.0721) (-33.1815, 27.0079) (-33.2581, 26.9462) knots 0 0 0 1 2 2 2
  spline S125 degree 2 poles (-33.2581, 26.9462) (-33.3445, 26.8795) (-33.4359, 26.6695) (-33.4359, 26.5139) knots 0 0 0 1 2 2 2
  spline S126 degree 2 poles (-33.4359, 26.5139) (-33.4359, 26.3608) (-33.3445, 26.1459) (-33.2556, 26.057) knots 0 0 0 1 2 2 2
  spline S127 degree 2 poles (-33.2556, 26.057) (-33.1642, 25.9705) (-32.9444, 25.8816) (-32.7987, 25.8692) knots 0 0 0 1 2 2 2
  line L192 (-32.7987, 25.8692) -> (-32.7987, 27.0771)
  line L193 (-33.2754, 29.0556) -> (-33.2754, 29.0358)
  spline S128 degree 2 poles (-33.2754, 29.0358) (-33.2877, 28.9913) (-33.2927, 28.895) (-33.2927, 28.8283) knots 0 0 0 1 2 2 2
  spline S129 degree 2 poles (-33.2927, 28.8283) (-33.2927, 28.6727) (-33.1568, 28.3664) (-33.0234, 28.2281) knots 0 0 0 1 2 2 2
  line L194 (-33.0234, 28.2281) -> (-31.4006, 28.2281)
  line L195 (-31.4006, 28.2281) -> (-31.4006, 27.8428)
  line L196 (-31.4006, 27.8428) -> (-33.6879, 27.8428)
  line L197 (-33.6879, 27.8428) -> (-33.6879, 28.2281)
  line L198 (-33.6879, 28.2281) -> (-33.347, 28.2281)
  spline S130 degree 2 poles (-33.347, 28.2281) (-33.5347, 28.4381) (-33.6879, 28.7518) (-33.6879, 28.9) knots 0 0 0 1 2 2 2
  spline S131 degree 2 poles (-33.6879, 28.9) (-33.6879, 28.9592) (-33.6829, 29.0185) (-33.6755, 29.0556) knots 0 0 0 1 2 2 2
  line L199 (-33.6755, 29.0556) -> (-33.2754, 29.0556)
  spline S132 degree 2 poles (-51.4024, 20.964) (-51.106, 20.964) (-50.6046, 20.764) (-50.4218, 20.5639) knots 0 0 0 1 2 2 2
  spline S133 degree 2 poles (-50.4218, 20.5639) (-50.239, 20.3663) (-50.039, 19.7735) (-50.039, 19.3882) knots 0 0 0 1 2 2 2
  spline S134 degree 2 poles (-50.039, 19.3882) (-50.039, 19.0053) (-50.2341, 18.4372) (-50.4194, 18.2272) knots 0 0 0 1 2 2 2
  spline S135 degree 2 poles (-50.4194, 18.2272) (-50.6021, 18.0222) (-51.1011, 17.8073) (-51.4098, 17.8073) knots 0 0 0 1 2 2 2
  spline S136 degree 2 poles (-51.4098, 17.8073) (-51.563, 17.8073) (-51.8322, 17.8518) (-51.9458, 17.8864) knots 0 0 0 1 2 2 2
  spline S137 degree 2 poles (-51.9458, 17.8864) (-52.0446, 17.9185) (-52.2496, 18.0099) (-52.3509, 18.0642) knots 0 0 0 1 2 2 2
  line L200 (-52.3509, 18.0642) -> (-52.3509, 18.5533)
  line L201 (-52.3509, 18.5533) -> (-52.3188, 18.5533)
  spline S138 degree 2 poles (-52.3188, 18.5533) (-52.2645, 18.5039) (-52.0965, 18.3656) (-51.9755, 18.2989) knots 0 0 0 1 2 2 2
  spline S139 degree 2 poles (-51.9755, 18.2989) (-51.8594, 18.2347) (-51.5852, 18.1531) (-51.4074, 18.1531) knots 0 0 0 1 2 2 2
  spline S140 degree 2 poles (-51.4074, 18.1531) (-51.2122, 18.1531) (-50.864, 18.3137) (-50.733, 18.4668) knots 0 0 0 1 2 2 2
  spline S141 degree 2 poles (-50.733, 18.4668) (-50.6046, 18.6224) (-50.4613, 19.0942) (-50.4613, 19.3882) knots 0 0 0 1 2 2 2
  spline S142 degree 2 poles (-50.4613, 19.3882) (-50.4613, 19.7018) (-50.612, 20.1539) (-50.7429, 20.3095) knots 0 0 0 1 2 2 2
  spline S143 degree 2 poles (-50.7429, 20.3095) (-50.8714, 20.4601) (-51.2147, 20.6133) (-51.4074, 20.6133) knots 0 0 0 1 2 2 2
  spline S144 degree 2 poles (-51.4074, 20.6133) (-51.5827, 20.6133) (-51.8816, 20.5268) (-51.9977, 20.4626) knots 0 0 0 1 2 2 2
  spline S145 degree 2 poles (-51.9977, 20.4626) (-52.1088, 20.3984) (-52.2743, 20.265) (-52.3213, 20.2181) knots 0 0 0 1 2 2 2
  line L202 (-52.3213, 20.2181) -> (-52.3509, 20.2181)
  line L203 (-52.3509, 20.2181) -> (-52.3509, 20.7022)
  spline S146 degree 2 poles (-52.3509, 20.7022) (-52.2496, 20.7491) (-52.0718, 20.8356) (-51.9458, 20.8751) knots 0 0 0 1 2 2 2
  spline S147 degree 2 poles (-51.9458, 20.8751) (-51.8124, 20.9196) (-51.5852, 20.964) (-51.4024, 20.964) knots 0 0 0 1 2 2 2
  spline S148 degree 2 poles (-54.5789, 19.7661) (-54.5789, 20.344) (-54.0231, 20.9739) (-53.5587, 20.9739) knots 0 0 0 1 2 2 2
  spline S149 degree 2 poles (-53.5587, 20.9739) (-53.082, 20.9739) (-52.5362, 20.3243) (-52.5362, 19.7661) knots 0 0 0 1 2 2 2
  spline S150 degree 2 poles (-52.5362, 19.7661) (-52.5362, 19.193) (-53.0993, 18.5582) (-53.5587, 18.5582) knots 0 0 0 1 2 2 2
  spline S151 degree 2 poles (-53.5587, 18.5582) (-54.0231, 18.5582) (-54.5789, 19.1906) (-54.5789, 19.7661) knots 0 0 0 1 2 2 2
  spline S152 degree 2 poles (-54.1812, 19.7661) (-54.1812, 19.3215) (-53.8576, 18.8892) (-53.5587, 18.8892) knots 0 0 0 1 2 2 2
  spline S153 degree 2 poles (-53.5587, 18.8892) (-53.2599, 18.8892) (-52.9338, 19.3215) (-52.9338, 19.7661) knots 0 0 0 1 2 2 2
  spline S154 degree 2 poles (-52.9338, 19.7661) (-52.9338, 20.1983) (-53.2599, 20.6429) (-53.5587, 20.6429) knots 0 0 0 1 2 2 2
  spline S155 degree 2 poles (-53.5587, 20.6429) (-53.8551, 20.6429) (-54.1812, 20.2057) (-54.1812, 19.7661) knots 0 0 0 1 2 2 2
  line L204 (-57.5676, 20.9097) -> (-57.5676, 19.5858)
  spline S156 degree 2 poles (-57.5676, 19.5858) (-57.5676, 19.4277) (-57.5429, 19.1584) (-57.5034, 19.0843) knots 0 0 0 1 2 2 2
  spline S157 degree 2 poles (-57.5034, 19.0843) (-57.4638, 19.0028) (-57.3132, 18.9238) (-57.1823, 18.9238) knots 0 0 0 1 2 2 2
  spline S158 degree 2 poles (-57.1823, 18.9238) (-57.0637, 18.9238) (-56.792, 19.0695) (-56.6487, 19.2078) knots 0 0 0 1 2 2 2
  spline S159 degree 2 poles (-56.6487, 19.2078) (-56.6512, 19.2424) (-56.6561, 19.3388) (-56.6561, 19.403) knots 0 0 0 1 2 2 2
  line L205 (-56.6561, 19.403) -> (-56.6561, 20.9097)
  line L206 (-56.6561, 20.9097) -> (-56.2708, 20.9097)
  line L207 (-56.2708, 20.9097) -> (-56.2708, 19.5858)
  spline S160 degree 2 poles (-56.2708, 19.5858) (-56.2708, 19.4277) (-56.2461, 19.1584) (-56.2066, 19.0843) knots 0 0 0 1 2 2 2
  spline S161 degree 2 poles (-56.2066, 19.0843) (-56.1671, 19.0028) (-56.0164, 18.9238) (-55.8855, 18.9238) knots 0 0 0 1 2 2 2
  spline S162 degree 2 poles (-55.8855, 18.9238) (-55.762, 18.9238) (-55.4878, 19.0794) (-55.3594, 19.2004) knots 0 0 0 1 2 2 2
  line L208 (-55.3594, 19.2004) -> (-55.3594, 20.9097)
  line L209 (-55.3594, 20.9097) -> (-54.9741, 20.9097)
  line L210 (-54.9741, 20.9097) -> (-54.9741, 18.6224)
  line L211 (-54.9741, 18.6224) -> (-55.3594, 18.6224)
  line L212 (-55.3594, 18.6224) -> (-55.3594, 18.8744)
  spline S163 degree 2 poles (-55.3594, 18.8744) (-55.5101, 18.7237) (-55.8065, 18.5582) (-55.9843, 18.5582) knots 0 0 0 1 2 2 2
  spline S164 degree 2 poles (-55.9843, 18.5582) (-56.1868, 18.5582) (-56.5005, 18.7435) (-56.582, 18.9534) knots 0 0 0 1 2 2 2
  spline S165 degree 2 poles (-56.582, 18.9534) (-56.7574, 18.7583) (-57.0884, 18.5582) (-57.2811, 18.5582) knots 0 0 0 1 2 2 2
  spline S166 degree 2 poles (-57.2811, 18.5582) (-57.4293, 18.5582) (-57.6713, 18.6496) (-57.7602, 18.7534) knots 0 0 0 1 2 2 2
  spline S167 degree 2 poles (-57.7602, 18.7534) (-57.8516, 18.8571) (-57.9529, 19.1683) (-57.9529, 19.403) knots 0 0 0 1 2 2 2
  line L213 (-57.9529, 19.403) -> (-57.9529, 20.9097)
  line L214 (-57.9529, 20.9097) -> (-57.5676, 20.9097)
  line L215 (-61.0874, 20.9097) -> (-61.0874, 19.5858)
  spline S168 degree 2 poles (-61.0874, 19.5858) (-61.0874, 19.4277) (-61.0627, 19.1584) (-61.0231, 19.0843) knots 0 0 0 1 2 2 2
  spline S169 degree 2 poles (-61.0231, 19.0843) (-60.9836, 19.0028) (-60.8329, 18.9238) (-60.702, 18.9238) knots 0 0 0 1 2 2 2
  spline S170 degree 2 poles (-60.702, 18.9238) (-60.5835, 18.9238) (-60.3118, 19.0695) (-60.1685, 19.2078) knots 0 0 0 1 2 2 2
  spline S171 degree 2 poles (-60.1685, 19.2078) (-60.171, 19.2424) (-60.1759, 19.3388) (-60.1759, 19.403) knots 0 0 0 1 2 2 2
  line L216 (-60.1759, 19.403) -> (-60.1759, 20.9097)
  line L217 (-60.1759, 20.9097) -> (-59.7906, 20.9097)
  line L218 (-59.7906, 20.9097) -> (-59.7906, 19.5858)
  spline S172 degree 2 poles (-59.7906, 19.5858) (-59.7906, 19.4277) (-59.7659, 19.1584) (-59.7264, 19.0843) knots 0 0 0 1 2 2 2
  spline S173 degree 2 poles (-59.7264, 19.0843) (-59.6869, 19.0028) (-59.5362, 18.9238) (-59.4053, 18.9238) knots 0 0 0 1 2 2 2
  spline S174 degree 2 poles (-59.4053, 18.9238) (-59.2818, 18.9238) (-59.0076, 19.0794) (-58.8792, 19.2004) knots 0 0 0 1 2 2 2
  line L219 (-58.8792, 19.2004) -> (-58.8792, 20.9097)
  line L220 (-58.8792, 20.9097) -> (-58.4938, 20.9097)
  line L221 (-58.4938, 20.9097) -> (-58.4938, 18.6224)
  line L222 (-58.4938, 18.6224) -> (-58.8792, 18.6224)
  line L223 (-58.8792, 18.6224) -> (-58.8792, 18.8744)
  spline S175 degree 2 poles (-58.8792, 18.8744) (-59.0298, 18.7237) (-59.3262, 18.5582) (-59.5041, 18.5582) knots 0 0 0 1 2 2 2
  spline S176 degree 2 poles (-59.5041, 18.5582) (-59.7066, 18.5582) (-60.0203, 18.7435) (-60.1018, 18.9534) knots 0 0 0 1 2 2 2
  spline S177 degree 2 poles (-60.1018, 18.9534) (-60.2772, 18.7583) (-60.6082, 18.5582) (-60.8008, 18.5582) knots 0 0 0 1 2 2 2
  spline S178 degree 2 poles (-60.8008, 18.5582) (-60.949, 18.5582) (-61.1911, 18.6496) (-61.28, 18.7534) knots 0 0 0 1 2 2 2
  spline S179 degree 2 poles (-61.28, 18.7534) (-61.3714, 18.8571) (-61.4727, 19.1683) (-61.4727, 19.403) knots 0 0 0 1 2 2 2
  line L224 (-61.4727, 19.403) -> (-61.4727, 20.9097)
  line L225 (-61.4727, 20.9097) -> (-61.0874, 20.9097)
  spline S180 degree 2 poles (-63.8933, 19.7661) (-63.8933, 20.344) (-63.3375, 20.9739) (-62.8732, 20.9739) knots 0 0 0 1 2 2 2
  spline S181 degree 2 poles (-62.8732, 20.9739) (-62.3965, 20.9739) (-61.8506, 20.3243) (-61.8506, 19.7661) knots 0 0 0 1 2 2 2
  spline S182 degree 2 poles (-61.8506, 19.7661) (-61.8506, 19.193) (-62.4138, 18.5582) (-62.8732, 18.5582) knots 0 0 0 1 2 2 2
  spline S183 degree 2 poles (-62.8732, 18.5582) (-63.3375, 18.5582) (-63.8933, 19.1906) (-63.8933, 19.7661) knots 0 0 0 1 2 2 2
  spline S184 degree 2 poles (-63.4956, 19.7661) (-63.4956, 19.3215) (-63.172, 18.8892) (-62.8732, 18.8892) knots 0 0 0 1 2 2 2
  spline S185 degree 2 poles (-62.8732, 18.8892) (-62.5743, 18.8892) (-62.2483, 19.3215) (-62.2483, 19.7661) knots 0 0 0 1 2 2 2
  spline S186 degree 2 poles (-62.2483, 19.7661) (-62.2483, 20.1983) (-62.5743, 20.6429) (-62.8732, 20.6429) knots 0 0 0 1 2 2 2
  spline S187 degree 2 poles (-62.8732, 20.6429) (-63.1696, 20.6429) (-63.4956, 20.2057) (-63.4956, 19.7661) knots 0 0 0 1 2 2 2
  line L226 (-66.0842, 20.9097) -> (-65.6989, 20.9097)
  line L227 (-65.6989, 20.9097) -> (-65.6989, 19.6055)
  spline S188 degree 2 poles (-65.6989, 19.6055) (-65.6989, 19.4474) (-65.6692, 19.1757) (-65.6248, 19.0942) knots 0 0 0 1 2 2 2
  spline S189 degree 2 poles (-65.6248, 19.0942) (-65.5778, 19.0078) (-65.4099, 18.9238) (-65.2666, 18.9238) knots 0 0 0 1 2 2 2
  spline S190 degree 2 poles (-65.2666, 18.9238) (-65.1234, 18.9238) (-64.8195, 19.0769) (-64.6738, 19.2004) knots 0 0 0 1 2 2 2
  line L228 (-64.6738, 19.2004) -> (-64.6738, 20.9097)
  line L229 (-64.6738, 20.9097) -> (-64.2885, 20.9097)
  line L230 (-64.2885, 20.9097) -> (-64.2885, 18.6224)
  line L231 (-64.2885, 18.6224) -> (-64.6738, 18.6224)
  line L232 (-64.6738, 18.6224) -> (-64.6738, 18.8769)
  spline S191 degree 2 poles (-64.6738, 18.8769) (-64.8467, 18.7212) (-65.1802, 18.5582) (-65.3679, 18.5582) knots 0 0 0 1 2 2 2
  spline S192 degree 2 poles (-65.3679, 18.5582) (-65.7038, 18.5582) (-66.0842, 19.0028) (-66.0842, 19.4252) knots 0 0 0 1 2 2 2
  line L233 (-66.0842, 19.4252) -> (-66.0842, 20.9097)
  spline S193 degree 2 poles (-52.9227, 26.0739) (-52.5991, 26.0739) (-52.0631, 25.8763) (-51.8705, 25.6763) knots 0 0 0 1 2 2 2
  spline S194 degree 2 poles (-51.8705, 25.6763) (-51.6778, 25.4737) (-51.4728, 24.876) (-51.4728, 24.4882) knots 0 0 0 1 2 2 2
  spline S195 degree 2 poles (-51.4728, 24.4882) (-51.4728, 24.1202) (-51.6803, 23.5372) (-51.873, 23.3297) knots 0 0 0 1 2 2 2
  spline S196 degree 2 poles (-51.873, 23.3297) (-52.0582, 23.1297) (-52.6016, 22.9123) (-52.9252, 22.9123) knots 0 0 0 1 2 2 2
  spline S197 degree 2 poles (-52.9252, 22.9123) (-53.0808, 22.9123) (-53.3624, 22.9568) (-53.4908, 22.9963) knots 0 0 0 1 2 2 2
  spline S198 degree 2 poles (-53.4908, 22.9963) (-53.5946, 23.0259) (-53.8465, 23.1346) (-53.9231, 23.1741) knots 0 0 0 1 2 2 2
  line L234 (-53.9231, 23.1741) -> (-53.9231, 23.6632)
  line L235 (-53.9231, 23.6632) -> (-53.8885, 23.6632)
  spline S199 degree 2 poles (-53.8885, 23.6632) (-53.8119, 23.5965) (-53.6514, 23.4755) (-53.5032, 23.4063) knots 0 0 0 1 2 2 2
  spline S200 degree 2 poles (-53.5032, 23.4063) (-53.3797, 23.3446) (-53.061, 23.2631) (-52.8783, 23.2631) knots 0 0 0 1 2 2 2
  spline S201 degree 2 poles (-52.8783, 23.2631) (-52.4386, 23.2631) (-51.8952, 23.925) (-51.8952, 24.4758) knots 0 0 0 1 2 2 2
  spline S202 degree 2 poles (-51.8952, 24.4758) (-51.8952, 24.7821) (-52.0384, 25.2415) (-52.1743, 25.3996) knots 0 0 0 1 2 2 2
  spline S203 degree 2 poles (-52.1743, 25.3996) (-52.3052, 25.5577) (-52.6757, 25.7232) (-52.9079, 25.7232) knots 0 0 0 1 2 2 2
  spline S204 degree 2 poles (-52.9079, 25.7232) (-53.0783, 25.7232) (-53.4192, 25.6738) (-53.5353, 25.6244) knots 0 0 0 1 2 2 2
  line L236 (-53.5353, 25.6244) -> (-53.5353, 24.8365)
  line L237 (-53.5353, 24.8365) -> (-52.8289, 24.8365)
  line L238 (-52.8289, 24.8365) -> (-52.8289, 24.4808)
  line L239 (-52.8289, 24.4808) -> (-53.9354, 24.4808)
  line L240 (-53.9354, 24.4808) -> (-53.9354, 25.8121)
  spline S205 degree 2 poles (-53.9354, 25.8121) (-53.8588, 25.8467) (-53.597, 25.9529) (-53.4859, 25.985) knots 0 0 0 1 2 2 2